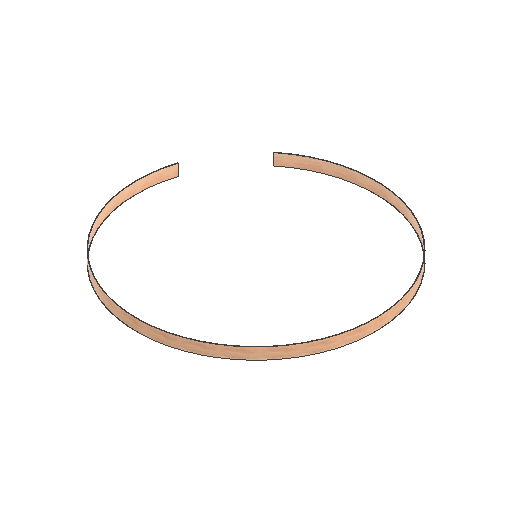
# Autodesk Inventor part: Edge Band - Platform B Outer
Saved by Autodesk Inventor 2021 (Build 250183000, 183)
## iProperties
Created: 2020-05-12
Part Number: Edge Band - Platform B Outer
Material: Wood (Birch)
Document SubType Name: Modeling
Designer: Dan Wikman
Density: 0.55 g/cm^3
Appearance: Birch - Natural Polished
Mass: 1295.24 g
Surface Area: 12254 cm^2
Volume: 2354.98 cm^3
Author: Dan Wikman
Autodesk Inventor part; units mm, degrees
ref_plane "YZ Plane" through (0, 0, 0) normal (1, 0, 0) x (0, 1, 0)
ref_plane "XZ Plane" through (0, 0, 0) normal (0, 1, 0) x (-1, 0, 0)
ref_plane "XY Plane" through (0, 0, 0) normal (0, 0, 1) x (1, 0, 0)
sketch "Sketch1" plane through (0, 0, 0) normal (0, 1, 0) x (-1, 0, 0)
  circle A0 centre (0, 0) radius 1031.19
  circle A1 centre (0, 0) radius 1035.19
  dimension "d0" = 2062.38
  dimension "d1" = 2070.38
  constraints: 2 centre point, 2 coincident
  measures "d0" diameter of A0
  measures "d1" diameter of A1
extrude "Extrusion1" add sketch "Sketch1" along normal blind 100
sketch "Sketch2" plane through (0, 0, 0) normal (0, -1, 0) x (1, 0, 0)
  line L0 (-983.2949, -310.6258) -> (-448.7923, -34.0427) projected
  line L1 (-195.6325, -404.1967) -> (-647.2539, -801.7903) projected
  line L2 (-659.5539, -812.6189) -> (-642.0164, -797.1795)
  circle A0 centre (0, 0) radius 1035.19 projected
  line L3 (-986.8982, -312.4904) -> (-983.2949, -310.6258)
  circle A1 centre (0, 0) radius 1031.19 projected
  point P0 (-647.8255, -802.2936)
  point P1 (-983.293, -310.6248)
  point P2 (-650.8713, -804.9751)
  constraints: 4 end point, 1 point on line, 2 other
extrude "Extrusion2" cut sketch "Sketch2" against normal blind 100 contours A0 L3 A1 L2 picked at (-659.8337, -793.9246)
body "Solid1"
